Autodesk Inventor part; units mm, degrees
(part 2 of 2)
  line L121 (-52.249, -25.9818) -> (-52.1484, -25.8612) construction
  spline S81 degree 3 poles (-52.1484, -25.8612) (-52.1393, -25.8923) (-52.1222, -25.9507) (-52.0938, -26.0317) (-52.0642, -26.1004) (-52.0328, -26.1565) (-52.0011, -26.2012) (-51.9675, -26.2331) (-51.9321, -26.2541) (-51.9071, -26.2568) (-51.8951, -26.258) knots 0 0 0 0 0.196044 0.368613 0.518981 0.648244 0.756985 0.848906 0.927701 1 1 1 1 construction
  spline S82 degree 3 poles (-51.8951, -26.258) (-51.8848, -26.2574) (-51.8642, -26.2563) (-51.8343, -26.2446) (-51.8052, -26.2274) (-51.7785, -26.2024) (-51.7525, -26.1728) (-51.731, -26.1369) (-51.7116, -26.0972) (-51.6963, -26.0529) (-51.684, -26.0057) (-51.6756, -25.9565) (-51.6701, -25.906) (-51.6693, -25.8718) (-51.669, -25.8545) knots 0 0 0 0 0.060787 0.122012 0.188076 0.26029 0.338632 0.420899 0.50789 0.601061 0.698616 0.797338 0.897017 1 1 1 1 construction
  spline S83 degree 3 poles (-51.669, -25.8545) (-51.6696, -25.8347) (-51.6709, -25.7951) (-51.6785, -25.7361) (-51.692, -25.6777) (-51.7049, -25.6399) (-51.7114, -25.6207) knots 0 0 0 0 0.248042 0.497848 0.745994 1 1 1 1 construction
  spline S84 degree 3 poles (-51.7114, -25.6207) (-51.7167, -25.6072) (-51.7276, -25.5791) (-51.7474, -25.5367) (-51.77, -25.4923) (-51.795, -25.4457) (-51.8235, -25.3972) (-51.8549, -25.3469) (-51.8892, -25.2943) (-51.9139, -25.2591) (-51.9265, -25.241) knots 0 0 0 0 0.099817 0.206658 0.320272 0.441749 0.569284 0.705431 0.848775 1 1 1 1 construction
  spline S85 degree 3 poles (-51.9265, -25.241) (-51.939, -25.2231) (-51.963, -25.1885) (-51.9967, -25.1384) (-52.0264, -25.0918) (-52.0526, -25.0493) (-52.0757, -25.0111) (-52.0944, -24.9763) (-52.1098, -24.9457) (-52.1179, -24.9261) (-52.1216, -24.9171) knots 0 0 0 0 0.17292 0.333592 0.478573 0.610332 0.728907 0.83203 0.923271 1 1 1 1 construction
  spline S86 degree 3 poles (-52.1216, -24.9171) (-52.132, -24.8889) (-52.1528, -24.8319) (-52.1725, -24.7423) (-52.1855, -24.6496) (-52.1871, -24.5866) (-52.188, -24.5546) knots 0 0 0 0 0.243404 0.490375 0.741031 1 1 1 1 construction
  spline S87 degree 3 poles (-52.188, -24.5546) (-52.1875, -24.5295) (-52.1868, -24.48) (-52.1789, -24.4076) (-52.1665, -24.3386) (-52.1498, -24.2735) (-52.1277, -24.2136) (-52.1026, -24.1593) (-52.0719, -24.1126) (-52.0386, -24.0721) (-52.0013, -24.0404) (-51.963, -24.0158) (-51.9217, -24.002) (-51.8937, -23.9999) (-51.8798, -23.9989) knots 0 0 0 0 0.10852 0.213444 0.313897 0.41114 0.503222 0.589199 0.668601 0.744106 0.814695 0.879097 0.939882 1 1 1 1 construction
  spline S88 degree 3 poles (-51.8798, -23.9989) (-51.865, -23.9999) (-51.8349, -24.002) (-51.7911, -24.0194) (-51.7496, -24.0476) (-51.717, -24.0788) (-51.6918, -24.1099) (-51.6717, -24.1382) (-51.6514, -24.171) (-51.6307, -24.2084) (-51.6106, -24.2506) (-51.5888, -24.2968) (-51.5676, -24.3478) (-51.5539, -24.3835) (-51.5468, -24.402) knots 0 0 0 0 0.079913 0.16289 0.251876 0.350704 0.406473 0.468935 0.539056 0.615875 0.700349 0.792574 0.892688 1 1 1 1 construction
  line L122 (-51.5468, -24.402) -> (-51.6432, -24.5484) construction
  spline S89 degree 3 poles (-51.6432, -24.5484) (-51.6492, -24.5334) (-51.6606, -24.5048) (-51.6783, -24.464) (-51.6955, -24.4277) (-51.711, -24.3947) (-51.7269, -24.3663) (-51.7415, -24.3413) (-51.7557, -24.3203) (-51.7732, -24.2984) (-51.7951, -24.2764) (-51.8236, -24.2573) (-51.8536, -24.2454) (-51.8743, -24.2439) (-51.8846, -24.2431) knots 0 0 0 0 0.117803 0.225513 0.324273 0.412093 0.491653 0.561993 0.623867 0.675945 0.767143 0.849316 0.925061 1 1 1 1 construction
  spline S90 degree 3 poles (-51.8846, -24.2431) (-51.8975, -24.244) (-51.9233, -24.2458) (-51.9589, -24.2644) (-51.9907, -24.2925) (-52.0171, -24.331) (-52.0388, -24.3766) (-52.0544, -24.4282) (-52.064, -24.4848) (-52.0652, -24.5242) (-52.0658, -24.5446) knots 0 0 0 0 0.099475 0.198092 0.304588 0.425591 0.556723 0.694657 0.842088 1 1 1 1 construction
  spline S91 degree 3 poles (-52.0658, -24.5446) (-52.0649, -24.5699) (-52.0631, -24.6202) (-52.053, -24.6829) (-52.0387, -24.7324) (-52.0255, -24.7713) (-52.008, -24.8114) (-51.9946, -24.8383) (-51.9876, -24.8523) knots 0 0 0 0 0.23681 0.470514 0.591024 0.718463 0.854358 1 1 1 1 construction
  spline S92 degree 3 poles (-51.9876, -24.8523) (-51.9851, -24.8569) (-51.9793, -24.8679) (-51.9675, -24.8857) (-51.9526, -24.9085) (-51.9341, -24.9357) (-51.9128, -24.968) (-51.8872, -25.0041) (-51.8587, -25.0453) (-51.8382, -25.0741) (-51.8273, -25.0893) knots 0 0 0 0 0.05519 0.130081 0.223898 0.340361 0.474847 0.629239 0.80397 1 1 1 1 construction
  spline S93 degree 3 poles (-51.8273, -25.0893) (-51.8143, -25.1082) (-51.789, -25.145) (-51.7537, -25.2001) (-51.7211, -25.2534) (-51.6921, -25.3053) (-51.6662, -25.3556) (-51.6431, -25.4041) (-51.6236, -25.4515) (-51.6014, -25.512) (-51.5799, -25.587) (-51.5603, -25.677) (-51.5492, -25.7674) (-51.5476, -25.8277) (-51.5468, -25.8578) knots 0 0 0 0 0.082521 0.160914 0.236026 0.30763 0.375315 0.439938 0.501364 0.55994 0.672229 0.782414 0.891558 1 1 1 1 construction
  spline S94 degree 3 poles (-51.5468, -25.8578) (-51.5471, -25.8791) (-51.5475, -25.9212) (-51.5526, -25.9831) (-51.5599, -26.043) (-51.5711, -26.1008) (-51.5847, -26.1567) (-51.602, -26.2101) (-51.622, -26.2615) (-51.6451, -26.3099) (-51.67, -26.3545) (-51.6966, -26.3939) (-51.7247, -26.4272) (-51.7545, -26.4541) (-51.7854, -26.4758) (-51.818, -26.4911) (-51.8521, -26.5008) (-51.8753, -26.5018) (-51.887, -26.5023) knots 0 0 0 0 0.080698 0.159198 0.235071 0.309226 0.381799 0.452629 0.521836 0.590509 0.655479 0.715263 0.769922 0.820223 0.866983 0.912231 0.955901 1 1 1 1 construction
  spline S95 degree 3 poles (-48.8177, -26.5023) (-48.8269, -26.5019) (-48.8453, -26.5013) (-48.8725, -26.4947) (-48.8988, -26.4842) (-48.9244, -26.4693) (-48.9499, -26.4515) (-48.9735, -26.428) (-48.997, -26.4012) (-49.0201, -26.3707) (-49.0412, -26.3356) (-49.0618, -26.2968) (-49.0816, -26.254) (-49.0985, -26.2065) (-49.1163, -26.156) (-49.1311, -26.1008) (-49.1454, -26.0418) (-49.159, -25.9784) (-49.171, -25.9097) (-49.1808, -25.8347) (-49.1893, -25.7533) (-49.1965, -25.6655) (-49.2015, -25.5712) (-49.2053, -25.4703) (-49.2077, -25.363) (-49.2081, -25.2894) (-49.2083, -25.2515) knots 0 0 0 0 0.01982 0.03942 0.059615 0.080377 0.102611 0.12624 0.151609 0.178882 0.208118 0.239383 0.2731 0.309131 0.347296 0.387992 0.431485 0.477488 0.52698 0.580981 0.639601 0.702538 0.769805 0.842131 0.918858 1 1 1 1 construction
  spline S96 degree 3 poles (-49.2083, -25.2515) (-49.2081, -25.2134) (-49.2076, -25.1393) (-49.2059, -25.0313) (-49.2022, -24.93) (-49.1962, -24.8354) (-49.19, -24.7475) (-49.1812, -24.6664) (-49.1714, -24.592) (-49.1599, -24.5237) (-49.1469, -24.4607) (-49.1328, -24.4021) (-49.1168, -24.3475) (-49.1005, -24.2965) (-49.0823, -24.2496) (-49.0628, -24.2067) (-49.0421, -24.1677) (-49.0205, -24.1325) (-48.9974, -24.1015) (-48.9742, -24.0739) (-48.9498, -24.051) (-48.9247, -24.032) (-48.899, -24.0171) (-48.8725, -24.0065) (-48.8453, -23.9999) (-48.8269, -23.9992) (-48.8177, -23.9989) knots 0 0 0 0 0.081717 0.158677 0.23125 0.298788 0.361617 0.419821 0.473415 0.522448 0.567988 0.611094 0.651502 0.689832 0.72562 0.759293 0.790516 0.820183 0.847694 0.873287 0.897132 0.919263 0.940463 0.960632 0.980205 1 1 1 1 construction
  spline S97 degree 3 poles (-48.8177, -23.9989) (-48.8082, -23.9992) (-48.7895, -23.9999) (-48.762, -24.0064) (-48.7353, -24.0172) (-48.7092, -24.032) (-48.6836, -24.0508) (-48.6592, -24.0741) (-48.6354, -24.1014) (-48.6122, -24.1329) (-48.5894, -24.1684) (-48.5689, -24.2086) (-48.5487, -24.2524) (-48.5301, -24.3006) (-48.5126, -24.3528) (-48.4965, -24.4094) (-48.4811, -24.4699) (-48.4674, -24.535) (-48.455, -24.605) (-48.4439, -24.6804) (-48.4351, -24.7616) (-48.4273, -24.8484) (-48.4219, -24.9411) (-48.4175, -25.0395) (-48.4152, -25.1437) (-48.4148, -25.215) (-48.4146, -25.2515) knots 0 0 0 0 0.02008 0.039931 0.060046 0.081483 0.103827 0.127608 0.153354 0.181265 0.211032 0.243231 0.277571 0.314018 0.353425 0.395123 0.439594 0.486812 0.537167 0.591382 0.649466 0.711503 0.777503 0.847857 0.921899 1 1 1 1 construction
  spline S98 degree 3 poles (-48.4146, -25.2515) (-48.4148, -25.2879) (-48.4152, -25.3589) (-48.4177, -25.4626) (-48.4212, -25.5605) (-48.4269, -25.6528) (-48.4346, -25.7391) (-48.4437, -25.8199) (-48.4538, -25.8951) (-48.4664, -25.9647) (-48.4803, -26.0293) (-48.495, -26.0896) (-48.5112, -26.146) (-48.5288, -26.1983) (-48.5472, -26.2467) (-48.5673, -26.2908) (-48.5887, -26.3308) (-48.611, -26.3668) (-48.6346, -26.3984) (-48.6586, -26.4262) (-48.6837, -26.4492) (-48.7089, -26.4686) (-48.735, -26.4838) (-48.7619, -26.4941) (-48.7894, -26.5015) (-48.8082, -26.502) (-48.8177, -26.5023) knots 0 0 0 0 0.077869 0.151673 0.221771 0.287523 0.349307 0.407133 0.461375 0.511465 0.558416 0.602537 0.644292 0.683754 0.720567 0.754955 0.787358 0.817453 0.845404 0.871665 0.895727 0.918305 0.939477 0.959935 0.979893 1 1 1 1 construction
  circle A11 centre (-65.4703, -28.8519) radius 7 construction
  line L123 (-29.4703, -18.8519) -> (-74.4703, -18.8519) construction
  line L124 (-74.4703, -18.8519) -> (-74.4703, -38.8519) construction
  line L125 (-74.4703, -38.8519) -> (-29.4703, -38.8519) construction
  line L126 (-29.4703, -38.8519) -> (-29.4703, -18.8519) construction
  point P0 (0, 0)
  point P1 (-49.1094, -27.0523)
  constraints: 254 end point, 12 centre point, 8 point on circle, 4 collinear, 2 parallel, 1 horizontal, 1 perpendicular, 202 other
extrude "Extrusion1" add sketch "Sketch1" along normal blind 9.169 contours A0 | A1 | L5 A3 L4 A2
body "Solid1"
